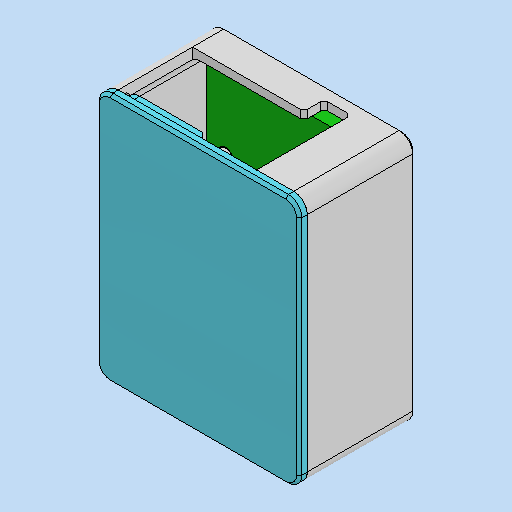
# Autodesk Inventor part: motorsplug
Saved by Autodesk Inventor 2025 (Build 290162000, 162)
## iProperties
Created: 2025-05-21
Part Number: motorsplug
Material: Generic
Document SubType Name: Modeling
Designer: kuzmin
Density: 1 g/cm^3
Appearance: Default
Author: kuzmin
Autodesk Inventor part; units mm, degrees
ref_plane "YZ Plane" through (0, 0, 0) normal (1, 0, 0) x (0, 1, 0)
ref_plane "XZ Plane" through (0, 0, 0) normal (0, 1, 0) x (-1, 0, 0)
ref_plane "XY Plane" through (0, 0, 0) normal (0, 0, 1) x (1, 0, 0)
sketch "Sketch1" plane through (0, 0, 0) normal (0, 0, 1) x (1, 0, 0)
  line L0 (-13, 16.5) -> (13, 16.5)
  line L1 (13, 16.5) -> (13, -16.5)
  line L2 (13, -16.5) -> (-13, -16.5)
  line L3 (-13, -16.5) -> (-13, 16.5)
  point P0 (0, 0)
  point P1 (13, 0)
  point P2 (0, 16.5)
  dimension "d0" = 26
  dimension "d1" = 33
  constraints: 8 end point, 2 midpoint, 2 parallel, 1 horizontal, 1 horizontal alignment, 1 perpendicular, 1 vertical alignment
  measures "d0" distance of L0.start L0.end
  measures "d1" distance of L0.end L1.end
extrude "Extrusion1" add sketch "Sketch1" along normal blind 2
sketch "Sketch2" plane through (0, 0, 2) normal (0, 0, 1) x (1, 0, 0)
  line L0 (-10.1, -5) -> (10.1, -5)
  line L1 (10.1, -5) -> (10.1, 5)
  line L2 (10.1, 5) -> (-10.1, 5)
  line L3 (-10.1, 5) -> (-10.1, -5)
  point P0 (0, 0)
  point P1 (0, 5)
  point P2 (-10.1, 0)
  dimension "d4" = 10
  dimension "d5" = 20.2
  constraints: 8 end point, 4 coincident, 2 midpoint, 2 parallel, 1 horizontal, 1 horizontal alignment, 1 perpendicular, 1 vertical alignment
  measures "d4" distance of L2.end L0.start
  measures "d5" distance of L1.end L2.end
hole "Hole1" at (-10.1, -5, 2) at (10.1, -5, 2) at (-10.1, 5, 2) at (10.1, 5, 2) direction (0, 0, -1) diameter 2.2 end through all
sketch "Sketch3" plane through (0, 0, 0) normal (0, 0, 1) x (1, 0, 0)
  line L0 (-15, 18.5) -> (15, 18.5)
  line L1 (15, 18.5) -> (15, -18.5)
  line L2 (15, -18.5) -> (-15, -18.5)
  line L3 (-15, -18.5) -> (-15, 18.5)
  point P0 (0, 0)
  point P1 (15, 0)
  point P2 (0, 18.5)
  dimension "d13" = 30
  dimension "d14" = 37
  constraints: 8 end point, 2 midpoint, 2 parallel, 1 horizontal, 1 horizontal alignment, 1 perpendicular, 1 vertical alignment
  measures "d13" distance of L0.start L0.end
  measures "d14" distance of L0.end L1.end
extrude "Extrusion2" add sketch "Sketch3" against normal blind 1 separate body
sketch "Sketch4" plane through (0, 0, 0) normal (0, 0, 1) x (1, 0, 0)
  circle A0 centre (-10.1, -5) radius 1.1 projected
  circle A1 centre (-10.1, 5) radius 1.1 projected
  circle A2 centre (10.1, 5) radius 1.1 projected
  circle A3 centre (10.1, -5) radius 1.1 projected
  circle A4 centre (-10.1, -5) radius 1
  circle A5 centre (-10.1, 5) radius 1
  circle A6 centre (10.1, 5) radius 1
  circle A7 centre (10.1, -5) radius 1
  point P0 (0, 0)
  dimension "d17" = 2
  constraints: 4 centre point, 4 coincident, 3 equal radius
  measures "d17" diameter of A4
extrude "Extrusion3" add sketch "Sketch4" along normal blind 4 contours A4 | A5 | A6 | A7 bodies 2
sketch "Sketch5" plane through (0, 0, 0) normal (0, 0, 1) x (1, 0, 0)
  line L0 (-13.8, 17.3) -> (13.8, 17.3)
  line L1 (13.8, 17.3) -> (13.8, -17.3)
  line L2 (13.8, -17.3) -> (-13.8, -17.3)
  line L3 (-13.8, -17.3) -> (-13.8, 17.3)
  line L4 (15, -18.5) -> (15, 18.5) projected
  line L5 (15, 18.5) -> (-15, 18.5) projected
  line L6 (-15, 18.5) -> (-15, -18.5) projected
  line L7 (-15, -18.5) -> (15, -18.5) projected
  point P0 (0, 0)
  point P1 (0, 17.3)
  point P2 (13.8, 0)
  dimension "d24" = 1.2
  dimension "d25" = 1.2
  constraints: 8 end point, 2 midpoint, 2 parallel, 1 horizontal, 1 horizontal alignment, 1 perpendicular, 1 vertical alignment
  measures "d24" distance between parallel lines of L4 L1
  measures "d25" distance between parallel lines of L5 L0
extrude "Extrusion4" add sketch "Sketch5" along normal blind 15 bodies 2
fillet "Fillet1" radius 2 8 edges at (-15, -18.5, 7) (15, -18.5, 7) (15, 18.5, 7) (-15, 18.5, 7) (-13.8, -17.3, 7.5) (13.8, -17.3, 7.5) (13.8, 17.3, 7.5) (-13.8, 17.3, 7.5)
chamfer "Chamfer2" distance 1 angle 45 8 edges at (0, 17.3, 0) (-13.2142, 16.7142, 0) (-13.8, 0, 0) (-13.2142, -16.7142, 0) (0, -17.3, 0) (13.2142, -16.7142, 0) (13.8, 0, 0) (13.2142, 16.7142, 0)
chamfer "Chamfer1" distance 2 angle 45 4 edges at (-11.1, -5, 0) (-11.1, 5, 0) (9.1, -5, 0) (9.1, 5, 0)
sketch "Sketch7" plane through (0, 0, 0) normal (0, 1, 0) x (-1, 0, 0)
  line L0 (13.2, 15) -> (14.4, 13.8)
  line L1 (14.4, 13.8) -> (13.2, 12.6)
  line L2 (13.2, 12.6) -> (13.2, 15)
  line L3 (13.8, 15) -> (13.8, 1) projected
  line L4 (13.8, 15) -> (15, 15) projected
  point P0 (0, 0)
  point P1 (13.2, 13.8)
  point P2 (13.8, 14.4)
  point P3 (13.8, 13.2)
  dimension "d34" = 90
  dimension "d35" = 0.6
  dimension "d36" = 1.2
  dimension "d37" = 1.2
  constraints: 6 end point, 1 horizontal alignment, 1 midpoint, 1 perpendicular, 1 vertical
  measures "d34" angle of L1 L0
  measures "d35" distance from line of L3 L0.end
  measures "d36" distance from line of L2 L0.end
  measures "d37" distance from line of L4 L0.end
sketch3d "3D Sketch1"
  arc A0 (-13.8, -15.3, 15) -> (-11.8, -17.3, 15) centre (-11.8, -15.3, 15) ccw
  line L0 (-11.8, -17.3, 15) -> (11.8, -17.3, 15)
  arc A1 (11.8, -17.3, 15) -> (13.8, -15.3, 15) centre (11.8, -15.3, 15) ccw
  line L1 (13.8, -15.3, 15) -> (13.8, 15.3, 15)
  arc A2 (13.8, 15.3, 15) -> (11.8, 17.3, 15) centre (11.8, 15.3, 15) ccw
  line L2 (11.8, 17.3, 15) -> (-11.8, 17.3, 15)
  arc A3 (-11.8, 17.3, 15) -> (-13.8, 15.3, 15) centre (-11.8, 15.3, 15) ccw
  line L3 (-13.8, 15.3, 15) -> (-13.8, -15.3, 15)
sweep "Sweep1" cut profiles "Sketch7" path "3D Sketch1" bodies 2
sketch "Sketch6" plane through (0, 0, 15) normal (0, 0, 1) x (1, 0, 0)
  line L0 (12.8, -6.3077) -> (12.8, -3.6923) projected
  line L1 (-13, -22.2291) -> (12.8, -22.2291)
  line L2 (12.8, -22.2291) -> (12.8, -13.2955)
  line L3 (12.8, -13.2955) -> (-13, -13.2955)
  line L4 (-13, -13.2955) -> (-13, -22.2291)
  line L5 (-13, 20.1351) -> (7.5, 20.1351)
  line L6 (7.5, 20.1351) -> (7.5, 14.2918)
  line L7 (7.5, 14.2918) -> (-13, 14.2918)
  line L8 (-13, 14.2918) -> (-13, 20.1351)
  line L9 (-13, 16.5) -> (-13, -16.5) projected
  line L10 (13, -16.5) -> (13, 16.5) projected
  point P0 (0, 0)
  point P1 (12.8, -15.3)
  point P2 (13, 16.5)
  point P3 (13, -16)
  dimension "d31" = 5.5
  constraints: 14 end point, 3 horizontal, 3 parallel, 3 point on line, 1 perpendicular, 1 vertical, 4 other
extrude "Extrusion5" cut sketch "Sketch6" against normal blind 11 contours L5 L6 L7 L8 bodies 2
sketch "Sketch8" plane through (-11.8, 17.3, 1) normal (0, -1, 0) x (1, 0, 0)
  line L0 (19.3, 12.2) -> (19.3, 3) projected
  line L1 (23.6, 0) -> (0, 0) projected
  line L2 (19.3, 3) -> (15.3, 3)
  line L3 (15.3, 3) -> (15.3, 0)
  line L4 (15.3, 0) -> (19.3, 0)
  line L5 (19.3, 0) -> (19.3, 3)
  point P0 (11.8, -1)
  point P1 (19.3, 0)
  dimension "d40" = 4
  constraints: 8 end point, 2 parallel, 1 horizontal, 1 perpendicular, 1 point on line
  measures "d40" distance of L0.end L2.end
extrude "Extrusion6" cut sketch "Sketch8" against normal through all bodies 2
chamfer "Chamfer3" distance 0.5 angle 45 3 edges at (7.5, 17.9, 1) (3.5, 17.9, 1) (3.5, 17.9, 4)
sketch "Sketch9" plane through (0, 0, 15) normal (0, 0, 1) x (1, 0, 0)
  arc A0 (-13, 18.5) -> (-15, 16.5) centre (-13, 16.5) ccw projected
  line L0 (-13, 18.5) -> (13, 18.5) projected
  arc A1 (15, 16.5) -> (13, 18.5) centre (13, 16.5) ccw projected
  line L1 (15, 16.5) -> (15, -16.5) projected
  arc A2 (13, -18.5) -> (15, -16.5) centre (13, -16.5) ccw projected
  line L2 (13, -18.5) -> (-13, -18.5) projected
  arc A3 (-15, -16.5) -> (-13, -18.5) centre (-13, -16.5) ccw projected
  line L3 (-15, -16.5) -> (-15, 16.5) projected
  point P0 (0, 0)
extrude "Extrusion7" add sketch "Sketch9" along normal blind 1.2 separate body
sketch "Sketch10" plane through (0, 0, 15) normal (0, 0, -1) x (-1, 0, 0)
  line L0 (-13.8, -15.3) -> (-13.8, 15.3) construction
  line L1 (-13.8, -15.3) -> (-13.8, 15.3) projected
  line L2 (13.8, 15.3) -> (13.8, -15.3) construction
  line L3 (13.8, 15.3) -> (13.8, -15.3) projected
  line L4 (-7.5, 17.3) -> (-7, 17.3) construction
  line L5 (-11.8, 17.3) -> (-7, 17.3) construction
  line L6 (-11.8, 17.3) -> (-7.5, 17.3) construction
  line L7 (-13.8, 17.3) -> (13.8, 17.3)
  line L8 (13.8, 17.3) -> (13.8, -17.3)
  line L9 (13.8, -17.3) -> (-13.8, -17.3)
  line L10 (-13.8, -17.3) -> (-13.8, 17.3)
  line L11 (12.6, 16.1) -> (-12.6, 16.1)
  line L12 (-12.6, 16.1) -> (-12.6, -16.1)
  line L13 (-12.6, -16.1) -> (12.6, -16.1)
  line L14 (12.6, -16.1) -> (12.6, 16.1)
  point P0 (0, 0)
  point P1 (13.8, 0)
  point P2 (0, 17.3)
  dimension "d48" = 1.2
  constraints: 16 end point, 4 parallel, 2 midpoint, 2 perpendicular, 2 point on line, 1 horizontal, 1 horizontal alignment, 1 vertical alignment, 3 other
  measures "d48" distance between parallel lines of L11 L7
extrude "Extrusion8" add sketch "Sketch10" along normal blind 2 bodies 3
fillet "Fillet2" radius 2 8 edges at (13.8, -17.3, 14) (12.6, -16.1, 14) (-13.8, -17.3, 14) (-12.6, -16.1, 14) (12.6, 16.1, 14) (13.8, 17.3, 14) (-13.8, 17.3, 14) (-12.6, 16.1, 14)
extrude "Extrusion9" add sketch "Sketch7" along normal mid plane 25 contours L0 L1 L3 bodies 3
sketch "Sketch11" plane through (0, 12.5, 0) normal (0, 1, 0) x (1, 0, 0)
  line L0 (-13.8, -13.2) -> (-14.4, -13.8) projected
  line L1 (-14.4, -13.8) -> (-13.8, -14.4) projected
  line L2 (-13.8, -13.2) -> (-13.8, -14.4) projected
  line L3 (-14.2586, -13.8) -> (-13.8, -13.3414)
  line L4 (-14.2586, -13.8) -> (-13.8, -14.2586)
  line L5 (-13.8, -15) -> (-13.8, -13) projected
  point P0 (0, 0)
  point P1 (-13.8, -14.2586)
  dimension "d54" = 0.1
  constraints: 4 end point, 2 point on line, 1 horizontal alignment, 1 parallel, 1 perpendicular
  measures "d54" distance between parallel lines of L3 L0
extrude "Extrusion10" cut sketch "Sketch11" against normal through all contours L2 L3 L4 L1 L0 bodies 3
chamfer "Chamfer4" distance 0.1 angle 45 1 edges at (-14.2586, 0, 13.8)
mirror "Mirror1" about plane through (0, 0, 0) normal (1, 0, 0) of "Extrusion10", "Chamfer4", "Extrusion9" bodies 3
fillet "Fillet3" radius 2 4 edges at (13.8, 12.5, 13.8) (13.8, -12.5, 13.8) (-13.8, -12.5, 13.8) (-13.8, 12.5, 13.8)
sketch "Sketch12" plane through (-11.8, 17.3, 15) normal (0, 1, 0) x (1, 0, 0)
  line L0 (1.2, 0) -> (22.4, 0) projected
  line L1 (10.3, 0) -> (21.3, 0)
  line L2 (21.3, 0) -> (21.3, 3.5026)
  line L3 (21.3, 3.5026) -> (10.3, 3.5026)
  line L4 (10.3, 3.5026) -> (10.3, 0)
  line L5 (19.3, 13.5) -> (19.3, 0) projected
  point P0 (11.8, 15)
  point P1 (10.3, 1.7513)
  point P2 (21.3, 0)
  dimension "d61" = 9
  dimension "d62" = 11
  constraints: 8 end point, 2 parallel, 1 horizontal, 1 midpoint, 1 perpendicular, 1 point on line
  measures "d61" distance from line of point (10.3, 1.751) L5
  measures "d62" distance of L2.end L3.end
extrude "Extrusion11" cut sketch "Sketch12" against normal up to surface (1.2 mm away) bodies 3
chamfer "Chamfer5" distance 1 angle 45 4 edges at (9.5, 16.7, 13) (-1.5, 16.7, 13) (9.5, 16.7, 15) (-1.5, 16.7, 15)
sketch "Sketch14" plane through (-13, -18.5, 15) normal (0, -1, 0) x (1, 0, 0)
  line L0 (0.5, -5) -> (25.5, -5)
  line L1 (25.5, -5) -> (25.5, -11)
  line L2 (25.5, -11) -> (0.5, -11)
  line L3 (0.5, -11) -> (0.5, -5)
  line L4 (26, -16) -> (0, -16) projected
  point P0 (13, -15)
  point P1 (13, -11)
  dimension "d73" = 25
  dimension "d74" = 5
  dimension "d75" = 6
  constraints: 8 end point, 2 parallel, 1 horizontal, 1 midpoint, 1 perpendicular, 1 vertical alignment
  measures "d73" distance of L0.start L0.end
  measures "d74" distance between parallel lines of L4 L2
  measures "d75" distance of L0.end L1.end
extrude "Extrusion13" cut sketch "Sketch14" against normal blind 4 bodies 2
chamfer "Chamfer6" distance 1 angle 45 4 edges at (12.5, -17.8367, 4) (12.5, -17.8367, 10) (-12.5, -17.8367, 10) (-12.5, -17.8367, 4)
chamfer "Chamfer7" distance 0.4 angle 45 8 edges at (15, 0, 16.2) (14.4142, 17.9142, 16.2) (0, 18.5, 16.2) (-14.4142, 17.9142, 16.2) (-15, 0, 16.2) (-14.4142, -17.9142, 16.2) (0, -18.5, 16.2) (14.4142, -17.9142, 16.2)
chamfer "Chamfer8" distance 0.4 angle 45 8 edges at (15, 0, -1) (14.4142, -17.9142, -1) (0, -18.5, -1) (-14.4142, -17.9142, -1) (-15, 0, -1) (-14.4142, 17.9142, -1) (0, 18.5, -1) (14.4142, 17.9142, -1)
equation "\"d24\" = wall"
equation "\"d25\" = wall"
equation "\"wall\" = 1.2"
body "Solid4"
